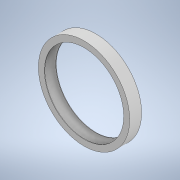
# Autodesk Inventor part: Part1
Saved by Autodesk Inventor 2022 (Build 260153000, 153)
## iProperties
Created: 2022-11-13
Part Number: Part1
Material: Generic
Document SubType Name: Modeling
Designer: trevo
Density: 1 g/cm^3
Appearance: Default
Author: trevo
Autodesk Inventor part; units mm, degrees
ref_plane "YZ Plane" through (0, 0, 0) normal (1, 0, 0) x (0, 1, 0)
ref_plane "XZ Plane" through (0, 0, 0) normal (0, 1, 0) x (-1, 0, 0)
ref_plane "XY Plane" through (0, 0, 0) normal (0, 0, 1) x (1, 0, 0)
sketch "Sketch1" plane through (0, 0, 0) normal (1, 0, 0) x (0, 1, 0)
  line L0 (0, 0) -> (0, -15.24)
  line L1 (0, -15.24) -> (7.62, -15.24)
  line L2 (0, 0) -> (7.62, 0)
  line L3 (7.62, 0) -> (7.62, -0.635)
  line L4 (7.62, -15.24) -> (7.62, -14.605)
  arc A0 (7.62, -0.635) -> (7.62, -14.605) centre (7.62, -7.62) ccw
  circle A1 centre (7.62, -7.62) radius 6.35 construction
  line L5 (0, 0) -> (-10.16, 0) construction
  line L6 (-10.16, 0) -> (-10.16, -15.24) construction
  line L7 (7.62, 0) -> (58.42, 0) construction
  line L8 (58.42, 0) -> (58.42, -15.24) construction
  dimension "d0" = 15.24
  dimension "d1" = 7.62
  dimension "d3" = 7.62
  dimension "d5" = 6.985
  dimension "d6" = 12.7
  dimension "d7" = 10.16
  dimension "d9" = 50.8
  constraints: 18 end point, 4 vertical, 3 horizontal, 2 centre point, 2 point on circle, 1 coincident, 1 perpendicular, 1 point on line
  measures "d0" distance of L0.start L0.end
  measures "d1" distance of L0.end L1.end
  measures "d3" distance of L0.start L2.end
  measures "d5" radius of A0
  measures "d6" diameter of A1
  measures "d7" distance of L0.start L5.end
  measures "d9" distance of L2.end L7.end
revolve "Revolution2" add sketch "Sketch1" angle 360 about axis through (0, 58.42, 0) along (0, 0, -1)
body "Solid2"
